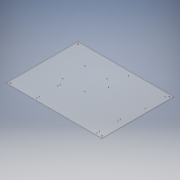
# Autodesk Inventor part: Acrylic_Mount
Saved by Autodesk Inventor 2019 (Build 230136000, 136)
## iProperties
Created: 2019-05-20
Part Number: Acrylic_Mount
Material: PET Plastic
Document SubType Name: Modeling
Designer: Jorian Bruslind
Density: 1.541 g/cm^3
Appearance: Polycarbonate - Clear
Author: Jorian Bruslind
Autodesk Inventor part; units mm, degrees
ref_plane "YZ Plane" through (0, 0, 0) normal (1, 0, 0) x (0, 1, 0)
ref_plane "XZ Plane" through (0, 0, 0) normal (0, 1, 0) x (-1, 0, 0)
ref_plane "XY Plane" through (0, 0, 0) normal (0, 0, 1) x (1, 0, 0)
sketch "Sketch1" plane through (0, 0, 0) normal (0, 1, 0) x (-1, 0, 0)
  line L0 (0, 0) -> (433, 0)
  line L1 (433, 0) -> (433, -325)
  line L2 (433, -325) -> (0, -325)
  line L3 (0, -325) -> (0, 0)
  dimension "d0" = 433
  dimension "d1" = 325
  constraints: 8 end point, 2 parallel, 1 horizontal, 1 perpendicular
  measures "d0" distance of L1.end L2.end
  measures "d1" distance of L0.end L1.end
extrude "Extrusion1" add sketch "Sketch1" along normal blind 3
sketch "Sketch2" plane through (0, 3, 0) normal (0, 1, 0) x (1, 0, 0)
  circle A0 centre (-10, 10) radius 2.75
  line L0 (0, 0) -> (0, 325) projected
  line L1 (-433, 0) -> (0, 0) projected
  circle A1 centre (-10, 315) radius 2.75
  circle A2 centre (-423, 10) radius 2.75
  circle A3 centre (-423, 315) radius 2.75
  dimension "d4" = 5.5
  dimension "d5" = 10
  dimension "d6" = 10
  dimension "d9" = 305
  dimension "d12" = 413
  constraints: 4 centre point, 1 horizontal, 1 vertical, 6 other
  measures "d4" diameter of A0
  measures "d5" distance from line of L0 A0.centre
  measures "d6" distance from line of L1 A0.centre
  measures "d9" distance of A0.centre A1.centre
  measures "d12" distance of A0.centre A2.centre
extrude "Extrusion2" cut sketch "Sketch2" against normal blind 3
sketch "Sketch5" plane through (0, 3, 0) normal (0, 1, 0) x (1, 0, 0)
  line L0 (0, 0) -> (0, 325) projected
  line L1 (0, 325) -> (0, 305)
  line L2 (0, 305) -> (-20, 305)
  circle A0 centre (-20, 305) radius 1.5
  line L3 (0, 325) -> (-433, 325) projected
  line L4 (0, 325) -> (-15, 325)
  circle A1 centre (-185, 305) radius 1.5
  circle A2 centre (-20, 215) radius 1.5
  circle A3 centre (-185, 215) radius 1.5
  dimension "d37" = 20
  dimension "d38" = 20
  dimension "d39" = 3
  dimension "d40" = 15
  dimension "d43" = 165
  dimension "d46" = 90
  constraints: 6 end point, 4 centre point, 2 point on line, 1 coincident, 1 horizontal, 1 perpendicular, 1 vertical, 6 other
  measures "d37" distance of L0.end L1.end
  measures "d38" distance of L1.end L2.end
  measures "d39" diameter of A0
  measures "d40" distance of L0.end L4.end
  measures "d43" distance of A0.centre A1.centre
  measures "d46" distance of A0.centre A2.centre
extrude "Extrusion5" cut sketch "Sketch5" against normal blind 3
sketch "Sketch6" plane through (0, 3, 0) normal (0, 1, 0) x (1, 0, 0)
  line L0 (-433, 0) -> (0, 0) projected
  line L1 (0, 0) -> (-33, 0)
  line L2 (-33, 0) -> (-33, 11)
  circle A0 centre (-33, 11) radius 1.5
  line L3 (-33, 11) -> (-33, 22)
  circle A1 centre (-33, 22) radius 1.5
  dimension "d51" = 33
  dimension "d52" = 11
  dimension "d53" = 3
  dimension "d54" = 11
  dimension "d55" = 180
  dimension "d56" = 3
  constraints: 6 end point, 2 centre point, 2 coincident, 1 point on line, 1 vertical
  measures "d51" distance of L0.end L1.end
  measures "d52" distance of L1.end L2.end
  measures "d53" diameter of A0
  measures "d54" distance of L3.start L3.end
  measures "d55" angle of L2 L3
  measures "d56" diameter of A1
extrude "Extrusion6" cut sketch "Sketch6" against normal blind 3
pattern_linear "Rectangular Pattern1" count 2 spacing 94 along (0, 0, -1) count 2 spacing 271.7 along (-1, 0, 0) of "Extrusion6"
sketch "Sketch7" plane through (0, 3, 0) normal (0, 1, 0) x (1, 0, 0)
  line L0 (-433, 325) -> (-433, 0) projected
  line L1 (-433, 325) -> (-322, 325)
  line L2 (0, 325) -> (-433, 325) projected
  line L3 (-322, 325) -> (-322, 245)
  circle A0 centre (-322, 245) radius 1.75
  circle A1 centre (-221.8, 245) radius 1.75
  circle A2 centre (-322, 144.8) radius 1.75
  circle A3 centre (-221.8, 144.8) radius 1.75
  point P0 (0, 0)
  dimension "d65" = 111
  dimension "d66" = 80
  dimension "d67" = 3.5
  dimension "d70" = 100.2
  dimension "d73" = 100.2
  constraints: 4 centre point, 4 end point, 2 vertical, 1 coincident, 1 horizontal, 1 point on line, 6 other
  measures "d65" distance of L0.start L1.end
  measures "d66" distance of L1.end L3.end
  measures "d67" diameter of A0
  measures "d70" distance of A0.centre A1.centre
  measures "d73" distance of A0.centre A2.centre
extrude "Extrusion7" cut sketch "Sketch7" against normal blind 3
body "Solid1"
